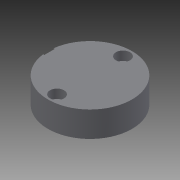
# Autodesk Inventor part: 02-2-0.13-FO1_BM_heads
Saved by Autodesk Inventor 2014 (Build 180170000, 170)
## iProperties
Category: PARTsolutions
Company: BIMBA
Created: 2014-01-19
Part Number: 02-2-0.13-FO1_BM_heads
Material: Generic
Catalog Web Link: www.cadenas.de
Description: FO1_basic_model_heads-Bimba FLAT-1
Vendor: BIMBA
Document SubType Name: Standard Catalog Part
Designer: Andrew Toennies
Manufacturer: BIMBA
Density: 1 g/cm^3
Appearance: RGB(211.00000262260440,211.00000262260440,211.00000262260440)
PSOL_IDENT_0: {$CADENAS_DATA\23d-libs\bimba\bimba\bimba_imperial\bimba_full_line\flat_cylinders\fo1\fo1_basic_mode
PSOL_IDENT_1: l_heads.prj},245 {VTYP=3D},{NB=02-2-0.13-FO1_BM_heads},{LINA=02-2-0.13-FO1_BM_heads},{NN=FO1_basic_m
PSOL_IDENT_2: odel_heads},{DATE=11.12.2012 11:54:33},{GEOMDATE=11.12.2012 12:54:00},{VERSION=},{LINEID=10},{LINESU
PSOL_IDENT_3: BID=-1},{WBVAR=MNT,LRR,ER,HD,STPT1,STPT2,STPT3,STPT4,PP,RL1}  {NB=02-2-0.13-FO1_BM_heads},{LINA=02-2
PSOL_IDENT_4: -0.13-FO1_BM_heads},{KT=DUMMY},{PN=02-2-0.13-FO1_BM_heads},{BORE=0.56250000},{BOREPN=02},{MNT=},{MNT
PSOL_IDENT_5: ALG='','Standard','1','Pivot Mount','1N','Pivot Mount 90 Deg. from Standard','3','Thraded Mounting H
PSOL_IDENT_6: oles','4','Screw Clearance Holes','5','Nose Mount'},{LRR=2},{ER=},{HD=},{STPT1=},{STPT2=},{STPT3=},{
PSOL_IDENT_7: STPT4=},{PP=},{PPALG='','Standard'},{A=1.12000000},{C=0.88000000},{AR=0.88000000},{DD=2.00000000},{D=
PSOL_IDENT_8: 0.11200000},{CPIL=0.12000000},{DC=0.18800000},{DCP=0.12000000},{DCD=0.85500000},{ES=0.16400000},{EC=
PSOL_IDENT_9: 0.00000000},{ED=0.46000000},{F=0.25000000},{H=0.22000000},{J=0.34},{J1=0.34000000},{K=0.14},{K1=0.14
PSOL_IDENT_10: 000000},{K2=0.27000000},{L=0.19000000},{LDP=0.20000000},{LP=0.16000000},{LPDP=0.28000000},{TD=0.6100
PSOL_IDENT_11: 0000},{TDDP=0.10000},{LSF=0.31250000},{LSFDP=0.02000000},{AA=0.06000000},{AB=0.75000000},{AC=0.38000
PSOL_IDENT_12: 000},{AD=0.50000000},{AD1=UNF},{AE=0.49750000},{AF=0.31000000},{M=0.00000000},{N=0.00000000},{P=0.00
PSOL_IDENT_13: 000000},{Q=0.19000000},{QQ=0.252},{R=0.11200000},{S=0.38000000},{T=0.19000000},{U=0.25000000},{W=0.7
PSOL_IDENT_14: 5000000},{X=0.17000000},{Y=0.63000000},{Z=0.19000000},{A13=0.11200000},{A14=0.16600000},{ANGLE=45.00
PSOL_IDENT_15: 000000},{JY=0.34},{JH=0.34},{PANGLE=0},{ANGLE1=45},{ANGLE11=45.00000000},{D11=0.12},{CONX=0.12000000
PSOL_IDENT_16: },{CONY=0.12000000},{G=0.29000000},{HH=0.54000000},{RD=0.24000000},{HDADD1=0.13000000},{HDADD=0},{GW=
PSOL_IDENT_17: 0.0775},{GD=0.4215},{GR=0.0315},{PW=0.0620},{PD=0.4975},{PR=0.0150},{RL1=0.13000}
CNS_NN: FO1_basic_model_heads
CNS_NT: Bimba FLAT-1
CNS_NB: 02-2-0.13-FO1_BM_heads
CNS_NBSYN: $PN.
CNS_LINA: 02-2-0.13-FO1_BM_heads
CNS_PN: 02-2-0.13-FO1_BM_heads
CNS_BORE: 9/16
CNS_BOREPN: 02
CNS_MNT: Standard
CNS_MNTALG: '','Standard','1','Pivot Mount','1N','Pivot Mount 90 Deg. from Standard','3','Thraded Mounting Holes','4','Screw Clearance Holes','5','Nose Mount'
CNS_LRR: 2
CNS_ER: Single Rod
CNS_HD: Standard Rear Head
CNS_STPT1: Without T1
CNS_STPT2: Without T2
CNS_STPT3: Without T3
CNS_STPT4: Without T4
CNS_PP: Standard
CNS_PPALG: '','Standard'
CNS_A: 1.12000000
CNS_C: 0.88000000
CNS_AR: 0.88000000
CNS_DD: 2.00000000
CNS_D: 0.11200000
CNS_CPIL: 0.12000000
CNS_DC: 0.18800000
CNS_DCP: 0.12000000
CNS_DCD: 0.85500000
CNS_ES: 0.16400000
CNS_EC: 0.00000000
CNS_ED: 0.46000000
CNS_F: 0.25000000
CNS_H: 0.22000000
CNS_J: 0.340
CNS_J1: 0.34000000
CNS_K: 0.140
CNS_K1: 0.14000000
CNS_K2: 0.27000000
CNS_L: 0.19000000
CNS_LDP: 0.20000000
CNS_LP: 0.16000000
CNS_LPDP: 0.28000000
CNS_TD: 0.61000000
CNS_TDDP: 0.10000
CNS_LSF: 0.31250000
CNS_LSFDP: 0.02000000
CNS_AA: 0.06000000
CNS_AB: 0.75000000
CNS_AC: 0.38000000
CNS_AD: 0.50000000
CNS_AD1: UNF
CNS_AE: 0.49750000
CNS_AF: 0.31000000
CNS_M: 0.00000000
CNS_N: 0.00000000
CNS_P: 0.00000000
CNS_Q: 0.19000000
CNS_QQ: 0.252
CNS_R: 0.11200000
CNS_S: 0.38000000
CNS_T: 0.19000000
CNS_U: 0.25000000
CNS_W: 0.75000000
CNS_X: 0.17000000
CNS_Y: 0.63000000
CNS_Z: 0.19000000
CNS_A13: 0.11200000
CNS_A14: 0.16600000
CNS_ANGLE: 45.00000000
CNS_JY: 0.340
CNS_JH: 0.340
CNS_PANGLE: 0.000
CNS_ANGLE1: 45.000
CNS_ANGLE11: 45.00000000
CNS_D11: 0.120
CNS_CONX: 0.12000000
CNS_CONY: 0.12000000
CNS_G: 0.29000000
CNS_HH: 0.54000000
CNS_RD: 0.24000000
CNS_HDADD1: 0.13000000
CNS_HDADD: 0.000
CNS_GW: 0.0775
CNS_GD: 0.4215
CNS_GR: 0.0315
CNS_PW: 0.0620
CNS_PD: 0.4975
CNS_PR: 0.0150
CNS_RL1: 0.13000
SUPPLIER: BIMBA
ARTICLENO: 02-2-0.13-FO1_BM_heads
BOMINFO: 02-2-0.13-FO1_BM_heads
CREATOR: CADENAS GmbH
Title: 02-2-0.13-FO1_BM_heads
Author: Cadenas PARTsolutions
Comments: Bimba FLAT-1
Autodesk Inventor part; units mm, degrees
ref_plane "YZ Plane" through (0, 0, 0) normal (1, 0, 0) x (0, 1, 0)
ref_plane "XZ Plane" through (0, 0, 0) normal (0, 1, 0) x (-1, 0, 0)
ref_plane "XY Plane" through (0, 0, 0) normal (0, 0, 1) x (1, 0, 0)
sketch "Sketch_1" plane through (0, 0, 0) normal (0, 0, 1) x (1, 0, 0)
  line L0 (0, 0) -> (0, 8.636)
  line L1 (0, 8.636) -> (14.224, 8.636)
  line L2 (14.224, 8.636) -> (14.224, 0)
  line L3 (14.224, 0) -> (0, 0)
  line L4 (0, 0) -> (0, 8.636)
  constraints: 10 end point
revolve "Revolution1" add sketch "Sketch_1" angle 360 about axis through (0, 0, 0) along (0, -1, 0)
sketch "Sketch_37" plane through (0, 0, 0) normal (0, 0, 1) x (1, 0, 0)
  line L0 (-5.9667, 5.08) -> (-14.224, 5.08)
  line L1 (-14.224, 5.08) -> (-14.224, 9.0488)
  line L2 (-14.224, 9.0488) -> (-13.716, 9.0488)
  line L3 (-13.716, 9.0488) -> (-13.716, 7.493)
  line L4 (-13.716, 7.493) -> (-13.2867, 7.0637)
  line L5 (-13.2867, 7.0637) -> (-7.112, 7.0637)
  line L6 (-7.112, 7.0637) -> (-5.9667, 5.08)
  line L7 (-5.9667, 5.08) -> (-14.224, 5.08)
  constraints: 16 end point
revolve "Revolution2" cut sketch "Sketch_37" angle 360 about axis through (-5.9667, 5.08, 0) along (1, 0, 0)
thread "Thread1" size "10-32 UNF" class "2B" standard "ANSI Unified Screw Threads" length 5.08 offset 1.524
sketch "Sketch3" plane through (0, 0, 0) normal (0, -1, 0) x (1, 0, 0)
  point P0 (0, 0)
hole "Hole1" at (0, 0, 0) direction (0, 1, 0) diameter 15.494 depth 2.54
sketch "Sketch4" plane through (0, 8.636, 0) normal (0, 1, 0) x (1, 0, 0)
  point P0 (0, -11.176)
hole "Hole2" at (0, 8.636, 11.176) direction (0, -1, 0) diameter 3.048 depth 8.636 counterbore diameter 4.7752 counterbore depth 3.048
sketch "Sketch5" plane through (0, 8.636, 0) normal (0, 1, 0) x (1, 0, 0)
  point P0 (0, 11.176)
hole "Hole3" at (0, 8.636, -11.176) direction (0, -1, 0) diameter 3.048 depth 8.636 counterbore diameter 4.7752 counterbore depth 3.048
sketch "Sketch6" plane through (0, 0, 0) normal (0, -1, 0) x (1, 0, 0)
  point P0 (-7.9026, 7.9026)
hole "Hole4" at (-7.9026, 0, 7.9026) direction (0, 1, 0) diameter 3.048 depth 2.54
sketch "Sketch7" plane through (0, 0, 0) normal (0, -1, 0) x (1, 0, 0)
  point P0 (7.9026, 7.9026)
hole "Hole5" at (7.9026, 0, 7.9026) direction (0, 1, 0) diameter 3.048 depth 2.54
sketch "Sketch8" plane through (0, 0, 0) normal (0, -1, 0) x (1, 0, 0)
  point P0 (7.9026, -7.9026)
hole "Hole6" at (7.9026, 0, -7.9026) direction (0, 1, 0) diameter 3.048 depth 2.54
sketch "Sketch9" plane through (0, 0, 0) normal (0, -1, 0) x (1, 0, 0)
  point P0 (-7.9026, -7.9026)
hole "Hole7" at (-7.9026, 0, -7.9026) direction (0, 1, 0) diameter 3.048 depth 2.54
ref_plane "a1_XY" through (0, 8.636, -14.224) normal (0, 1, 0) x (1, 0, 0)
ref_plane "a1_YZ" through (0, 8.636, -14.224) normal (1, 0, 0) x (0, 0, -1)
ref_plane "a1_ZX" through (0, 8.636, -14.224) normal (0, 0, -1) x (0, 1, 0)
ref_plane "a2_XY" through (0, 8.636, 14.224) normal (0, 1, 0) x (1, 0, 0)
ref_plane "a2_YZ" through (0, 8.636, 14.224) normal (1, 0, 0) x (0, 0, -1)
ref_plane "a2_ZX" through (0, 8.636, 14.224) normal (0, 0, -1) x (0, 1, 0)
ref_plane "ar3_XY" through (-7.9026, 2.54, 7.9026) normal (0, 1, 0) x (1, 0, 0)
ref_plane "ar3_YZ" through (-7.9026, 2.54, 7.9026) normal (1, 0, 0) x (0, 0, -1)
ref_plane "ar3_ZX" through (-7.9026, 2.54, 7.9026) normal (0, 0, -1) x (0, 1, 0)
ref_plane "ar4_XY" through (7.9026, 2.54, 7.9026) normal (0, 1, 0) x (1, 0, 0)
ref_plane "ar4_YZ" through (7.9026, 2.54, 7.9026) normal (1, 0, 0) x (0, 0, -1)
ref_plane "ar4_ZX" through (7.9026, 2.54, 7.9026) normal (0, 0, -1) x (0, 1, 0)
ref_plane "ar5_XY" through (7.9026, 2.54, -7.9026) normal (0, 1, 0) x (1, 0, 0)
ref_plane "ar5_YZ" through (7.9026, 2.54, -7.9026) normal (1, 0, 0) x (0, 0, -1)
ref_plane "ar5_ZX" through (7.9026, 2.54, -7.9026) normal (0, 0, -1) x (0, 1, 0)
ref_plane "ar6_XY" through (-7.9026, 2.54, -7.9026) normal (0, 1, 0) x (1, 0, 0)
ref_plane "ar6_YZ" through (-7.9026, 2.54, -7.9026) normal (1, 0, 0) x (0, 0, -1)
ref_plane "ar6_ZX" through (-7.9026, 2.54, -7.9026) normal (0, 0, -1) x (0, 1, 0)
ref_plane "b1_XY" through (0, 8.636, 0) normal (0, 1, 0) x (1, 0, 0)
ref_plane "b1_YZ" through (0, 8.636, 0) normal (1, 0, 0) x (0, 0, -1)
ref_plane "b1_ZX" through (0, 8.636, 0) normal (0, 0, -1) x (0, 1, 0)
ref_plane "c1_XY" through (0, 8.636, -11.176) normal (0, 1, 0) x (1, 0, 0)
ref_plane "c1_YZ" through (0, 8.636, -11.176) normal (1, 0, 0) x (0, 0, -1)
ref_plane "c1_ZX" through (0, 8.636, -11.176) normal (0, 0, -1) x (0, 1, 0)
ref_plane "c2_XY" through (0, 8.636, 11.176) normal (0, 1, 0) x (1, 0, 0)
ref_plane "c2_YZ" through (0, 8.636, 11.176) normal (1, 0, 0) x (0, 0, -1)
ref_plane "c2_ZX" through (0, 8.636, 11.176) normal (0, 0, -1) x (0, 1, 0)
ref_plane "d1_XY" through (-1.524, 8.636, -11.176) normal (0, 1, 0) x (1, 0, 0)
ref_plane "d1_YZ" through (-1.524, 8.636, -11.176) normal (1, 0, 0) x (0, 0, -1)
ref_plane "d1_ZX" through (-1.524, 8.636, -11.176) normal (0, 0, -1) x (0, 1, 0)
ref_plane "d2_XY" through (1.524, 8.636, -11.176) normal (0, 1, 0) x (1, 0, 0)
ref_plane "d2_YZ" through (1.524, 8.636, -11.176) normal (1, 0, 0) x (0, 0, -1)
ref_plane "d2_ZX" through (1.524, 8.636, -11.176) normal (0, 0, -1) x (0, 1, 0)
ref_plane "j_XY" through (0, 0, 0) normal (0, 1, 0) x (1, 0, 0)
ref_plane "j_YZ" through (0, 0, 0) normal (1, 0, 0) x (0, 0, -1)
ref_plane "j_ZX" through (0, 0, 0) normal (0, 0, -1) x (0, 1, 0)
ref_plane "k1_XY" through (-14.224, 5.08, 0) normal (0, 0, 1) x (1, 0, 0)
ref_plane "k1_YZ" through (-14.224, 5.08, 0) normal (1, 0, 0) x (0, 1, 0)
ref_plane "k1_ZX" through (-14.224, 5.08, 0) normal (0, 1, 0) x (0, 0, 1)
ref_plane "k2_XY" through (-14.224, 8.636, 0) normal (0, 0, 1) x (1, 0, 0)
ref_plane "k2_YZ" through (-14.224, 8.636, 0) normal (1, 0, 0) x (0, 1, 0)
ref_plane "k2_ZX" through (-14.224, 8.636, 0) normal (0, 1, 0) x (0, 0, 1)
ref_plane "l1_XY" through (-14.224, 7.493, 0) normal (0, 0, 1) x (1, 0, 0)
ref_plane "l1_YZ" through (-14.224, 7.493, 0) normal (1, 0, 0) x (0, 1, 0)
ref_plane "l1_ZX" through (-14.224, 7.493, 0) normal (0, 1, 0) x (0, 0, 1)
ref_plane "l2_XY" through (-14.224, 2.667, 0) normal (0, 0, 1) x (1, 0, 0)
ref_plane "l2_YZ" through (-14.224, 2.667, 0) normal (1, 0, 0) x (0, 1, 0)
ref_plane "l2_ZX" through (-14.224, 2.667, 0) normal (0, 1, 0) x (0, 0, 1)
ref_plane "rg_XY" through (0, 8.636, 0) normal (0, 1, 0) x (1, 0, 0)
ref_plane "rg_YZ" through (0, 8.636, 0) normal (1, 0, 0) x (0, 0, -1)
ref_plane "rg_ZX" through (0, 8.636, 0) normal (0, 0, -1) x (0, 1, 0)
ref_plane "rh_XY" through (0, 8.636, 0) normal (0, 1, 0) x (1, 0, 0)
ref_plane "rh_YZ" through (0, 8.636, 0) normal (1, 0, 0) x (0, 0, -1)
ref_plane "rh_ZX" through (0, 8.636, 0) normal (0, 0, -1) x (0, 1, 0)
ref_plane "to_dummy_XY" through (0, 8.636, 0) normal (0, 1, 0) x (1, 0, 0)
ref_plane "to_dummy_YZ" through (0, 8.636, 0) normal (1, 0, 0) x (0, 0, -1)
ref_plane "to_dummy_ZX" through (0, 8.636, 0) normal (0, 0, -1) x (0, 1, 0)
ref_plane "to_nut_XY" through (0, 10.16, 0) normal (0, 1, 0) x (1, 0, 0)
ref_plane "to_nut_YZ" through (0, 10.16, 0) normal (1, 0, 0) x (0, 0, -1)
ref_plane "to_nut_ZX" through (0, 10.16, 0) normal (0, 0, -1) x (0, 1, 0)
ref_plane "to_rod_XY" through (0, 8.636, 0) normal (0, 1, 0) x (1, 0, 0)
ref_plane "to_rod_YZ" through (0, 8.636, 0) normal (1, 0, 0) x (0, 0, -1)
ref_plane "to_rod_ZX" through (0, 8.636, 0) normal (0, 0, -1) x (0, 1, 0)
ref_plane "to_tube_XY" through (0, 2.54, 0) normal (0, 1, 0) x (1, 0, 0)
ref_plane "to_tube_YZ" through (0, 2.54, 0) normal (1, 0, 0) x (0, 0, -1)
ref_plane "to_tube_ZX" through (0, 2.54, 0) normal (0, 0, -1) x (0, 1, 0)
ref_plane "to_wiper_XY" through (0, 8.636, 0) normal (0, 1, 0) x (1, 0, 0)
ref_plane "to_wiper_YZ" through (0, 8.636, 0) normal (1, 0, 0) x (0, 0, -1)
ref_plane "to_wiper_ZX" through (0, 8.636, 0) normal (0, 0, -1) x (0, 1, 0)
ref_plane "track1_XY" through (-7.874, 0, 0) normal (0, 1, 0) x (1, 0, 0)
ref_plane "track1_YZ" through (-7.874, 0, 0) normal (1, 0, 0) x (0, 0, -1)
ref_plane "track1_ZX" through (-7.874, 0, 0) normal (0, 0, -1) x (0, 1, 0)
ref_plane "track2_XY" through (0, 0, -7.874) normal (0, 1, 0) x (1, 0, 0)
ref_plane "track2_YZ" through (0, 0, -7.874) normal (1, 0, 0) x (0, 0, -1)
ref_plane "track2_ZX" through (0, 0, -7.874) normal (0, 0, -1) x (0, 1, 0)
ref_plane "track3_XY" through (7.874, 0, 0) normal (0, 1, 0) x (1, 0, 0)
ref_plane "track3_YZ" through (7.874, 0, 0) normal (1, 0, 0) x (0, 0, -1)
ref_plane "track3_ZX" through (7.874, 0, 0) normal (0, 0, -1) x (0, 1, 0)
ref_plane "track4_XY" through (0, 0, 7.874) normal (0, 1, 0) x (1, 0, 0)
ref_plane "track4_YZ" through (0, 0, 7.874) normal (1, 0, 0) x (0, 0, -1)
ref_plane "track4_ZX" through (0, 0, 7.874) normal (0, 0, -1) x (0, 1, 0)
body "Solid1"
